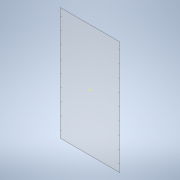
# Autodesk Inventor part: SP25V1 Acrilico
Saved by Autodesk Inventor 2021.2 (Build 252289000, 289)
## iProperties
Created: 2026-06-02
Part Number: SP25V1 Acrilico
Material: Cristal
Document SubType Name: Modeling
Designer: nelso
Density: 2.18 g/cm^3
Appearance: Transparente - Claro
Mass: 9370.9 g
Surface Area: 28808.3 cm^2
Volume: 4298.58 cm^3
Author: nelso
Autodesk Inventor part; units mm, degrees
ref_plane "YZ Plane" through (0, 0, 0) normal (1, 0, 0) x (0, 1, 0)
ref_plane "XZ Plane" through (0, 0, 0) normal (0, 1, 0) x (-1, 0, 0)
ref_plane "XY Plane" through (0, 0, 0) normal (0, 0, 1) x (1, 0, 0)
sketch "Sketch1" plane through (0, 0, 0) normal (0, 0, 1) x (1, 0, 0)
  line L0 (-434.2, -825) -> (434.2, -825)
  line L1 (434.2, -825) -> (434.2, 825)
  line L2 (434.2, 825) -> (-434.2, 825)
  line L3 (-434.2, 825) -> (-434.2, -825)
  line L4 (-434.2, -825) -> (434.2, 825) construction
  line L5 (434.2, -825) -> (-434.2, 825) construction
  point P0 (0, 0)
  dimension "d0" = 868.4
  dimension "d1" = 1650
  constraints: 12 end point, 2 midpoint, 2 parallel, 1 horizontal, 1 perpendicular
  measures "d0" distance of L2.end L1.end
  measures "d1" distance of L1.end L0.end
extrude "Extrusion1" add sketch "Sketch1" along normal blind 3
sketch "Sketch2" plane through (0, 0, 3) normal (0, 0, 1) x (1, 0, 0)
  point P0 (0, 0)
sketch "Sketch3" plane through (0, 0, 3) normal (0, 0, 1) x (1, 0, 0)
  circle A0 centre (420.85, -720) radius 2.25 projected
  circle A1 centre (420.85, -540) radius 2.25 projected
  circle A2 centre (420.85, -360) radius 2.25 projected
  circle A3 centre (420.85, -180) radius 2.25 projected
  circle A4 centre (420.85, 0) radius 2.25 projected
  circle A5 centre (420.85, 180) radius 2.25 projected
  circle A6 centre (420.85, 360) radius 2.25 projected
  circle A7 centre (420.85, 540) radius 2.25 projected
  circle A8 centre (420.85, 720) radius 2.25 projected
  circle A9 centre (-420.85, -720) radius 2.25 projected
  circle A10 centre (-420.85, -540) radius 2.25 projected
  circle A11 centre (-420.85, -360) radius 2.25 projected
  circle A12 centre (-420.85, -180) radius 2.25 projected
  circle A13 centre (-420.85, 0) radius 2.25 projected
  circle A14 centre (-420.85, 180) radius 2.25 projected
  circle A15 centre (-420.85, 360) radius 2.25 projected
  circle A16 centre (-420.85, 540) radius 2.25 projected
  circle A17 centre (-420.85, 720) radius 2.25 projected
  point P0 (0, 0)
extrude "Extrusion2" cut sketch "Sketch3" against normal blind 10
body "Solid1"
